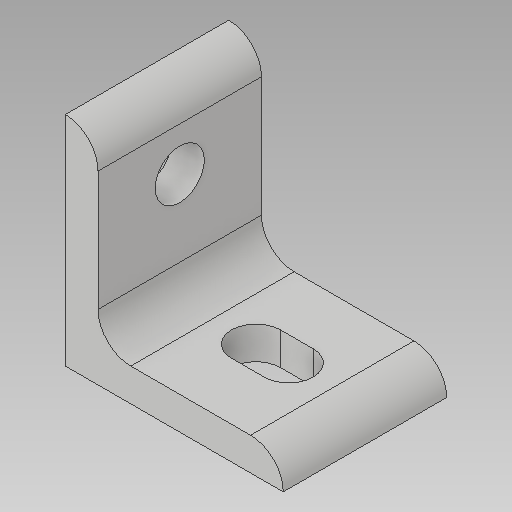
# Autodesk Inventor part: M4L
Saved by Autodesk Inventor 2021.2 (Build 252289000, 289)
## iProperties
Created: 2017-07-19
Part Number: M4L
Material: 一般
Document SubType Name: Modeling
Designer: gisen
Density: 1 g/cm^3
Appearance: 既定
Author: gisen
Autodesk Inventor part; units mm, degrees
ref_plane "YZ Plane" through (0, 0, 0) normal (1, 0, 0) x (0, 1, 0)
ref_plane "XZ Plane" through (0, 0, 0) normal (0, 1, 0) x (-1, 0, 0)
ref_plane "XY Plane" through (0, 0, 0) normal (0, 0, 1) x (1, 0, 0)
sketch "スケッチ1" plane through (0, 0, 0) normal (0, 0, 1) x (1, 0, 0)
  line L0 (0, 0) -> (0, 20)
  line L1 (0, 20) -> (3, 20)
  line L2 (3, 20) -> (3, 3)
  line L3 (3, 3) -> (20, 3)
  line L4 (20, 3) -> (20, 0)
  line L5 (20, 0) -> (0, 0)
  dimension "d0" = 3
  dimension "d1" = 3
  dimension "d2" = 20
  dimension "d3" = 20
  constraints: 12 end point, 5 perpendicular, 1 vertical
  measures "d0" distance of L0.end L1.end
  measures "d1" distance of L3.end L4.end
  measures "d2" distance of L0.start L0.end
  measures "d3" distance of L4.end L0.start
extrude "押し出し1" add sketch "スケッチ1" along normal blind 15
fillet "フィレット1" radius 3 2 edges at (3, 20, 7.5) (20, 3, 7.5)
sketch "スケッチ2" plane through (0, 0, 0) normal (-1, 0, 0) x (0, 0, 1)
  line L0 (0, 0) -> (0, 20) construction
  line L1 (0, 0) -> (15, 0) construction
  line L2 (15, 20) -> (15, 0) construction
  line L3 (0, 20) -> (15, 20) construction
  circle A0 centre (7.5, 13) radius 2.25
  dimension "d7" = 13
  dimension "d8" = 4.5
  dimension "d9" = 7.5
  constraints: 1 centre point
  measures "d7" distance from line of L1 A0.centre
  measures "d8" diameter of A0
  measures "d9" distance from line of L0 A0.centre
extrude "押し出し2" cut sketch "スケッチ2" against normal through all
sketch "スケッチ3" plane through (0, 0, 0) normal (0, -1, 0) x (1, 0, 0)
  arc A0 (10, 9.75) -> (10, 5.25) centre (10, 7.5) ccw
  line L0 (10, 7.5) -> (10, 9.75) construction
  line L1 (10, 7.5) -> (12.25, 7.5) construction
  line L2 (10, 7.5) -> (10, 5.25) construction
  arc A1 (13, 5.25) -> (13, 9.75) centre (13, 7.5) ccw
  line L3 (13, 7.5) -> (13, 9.75) construction
  line L4 (13, 7.5) -> (15.25, 7.5) construction
  line L5 (13, 7.5) -> (13, 5.25) construction
  line L6 (10, 9.75) -> (13, 9.75)
  line L7 (0, 15) -> (20, 15) projected
  line L8 (13, 5.25) -> (10, 5.25)
  line L9 (0, 0) -> (0, 15) projected
  dimension "d12" = 90
  dimension "d13" = 180
  dimension "d14" = 90
  dimension "d15" = 180
  dimension "d16" = 7.5
  dimension "d17" = 3
  dimension "d18" = 10
  dimension "d19" = 2.25
  constraints: 16 end point, 5 point on circle, 2 centre point, 2 horizontal, 2 parallel, 2 perpendicular, 1 tangent
  measures "d12" angle of L1 L0
  measures "d13" angle of L2 L0
  measures "d14" angle of L4 L3
  measures "d15" angle of L3 L5
  measures "d16" distance between parallel lines of L4 L7
  measures "d17" distance of L0.start L3.start
  measures "d18" distance from line of L9 L0.start
  measures "d19" radius of A1
extrude "押し出し3" cut sketch "スケッチ3" against normal through all
fillet "フィレット2" radius 3 1 edges at (3, 3, 7.5)
